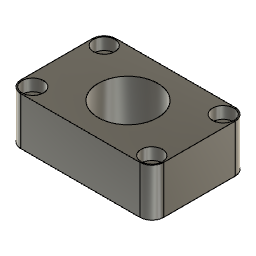
Complete Blueprint - Challenge (Autodesk Fusion 360 design; units mm, degrees)
Autodesk Fusion 360 part; units mm, degrees
sketch "Sketch1" plane through (0, 0, 0) normal (0, 0, 1) x (1, 0, 0)
  line L0 (38.1, -25.4) -> (-38.1, -25.4)
  line L1 (-38.1, -25.4) -> (-38.1, 25.4)
  line L2 (-38.1, 25.4) -> (38.1, 25.4)
  line L3 (38.1, 25.4) -> (38.1, -25.4)
  line L4 (38.1, -25.4) -> (-38.1, 25.4) construction
  line L5 (-38.1, -25.4) -> (38.1, 25.4) construction
  circle A0 centre (0, 0) radius 15.875
  dimension "d1" = 76.2
  dimension "d2" = 50.8
  dimension "d3" = 31.75
  constraint horizontal L0
  constraint perpendicular L0 L1
  constraint parallel L0 L2
  constraint parallel L1 L3
  constraint coincident L4 A0.centre
  constraint coincident L5 A0.centre
  constraint coincident A0.centre origin
  measures "d1" distance of L1.end L2.end
  measures "d2" distance of L0.end L1.end
  measures "d3" diameter of A0
extrude "Extrude1" add sketch "Sketch1" along normal blind 25.4
fillet "Fillet1" radius 6.35 4 edges at (38.1, 25.4, 12.7) (38.1, -25.4, 12.7) (-38.1, -25.4, 12.7) (-38.1, 25.4, 12.7)
sketch "Sketch2" plane through (0, 0, 25.4) normal (0, 0, 1) x (-1, 0, 0)
  circle A0 centre (0, 0) radius 15.875
  arc A1 (31.75, -25.4) -> (38.1, -19.05) centre (31.75, -19.05) ccw
  line L0 (38.1, -19.05) -> (38.1, 19.05)
  arc A2 (38.1, 19.05) -> (31.75, 25.4) centre (31.75, 19.05) ccw
  line L1 (31.75, 25.4) -> (-31.75, 25.4)
  arc A3 (-31.75, 25.4) -> (-38.1, 19.05) centre (-31.75, 19.05) ccw
  line L2 (-38.1, 19.05) -> (-38.1, -19.05)
  arc A4 (-38.1, -19.05) -> (-31.75, -25.4) centre (-31.75, -19.05) ccw
  line L3 (-31.75, -25.4) -> (31.75, -25.4)
  point P0 (31.75, -19.05)
  point P1 (-31.75, -19.05)
  point P2 (-31.75, 19.05)
  point P3 (31.75, 19.05)
  constraint coincident P0 A1.centre
  constraint coincident P1 A4.centre
  constraint coincident P2 A3.centre
  constraint coincident P3 A2.centre
hole "Hole1" at (-31.75, 19.05, 25.4) at (-31.75, -19.05, 25.4) at (31.75, -19.05, 25.4) at (31.75, 19.05, 25.4) direction (0, 0, -1) diameter 6.604 end through all counterbore diameter 11.43 counterbore depth 6.35
